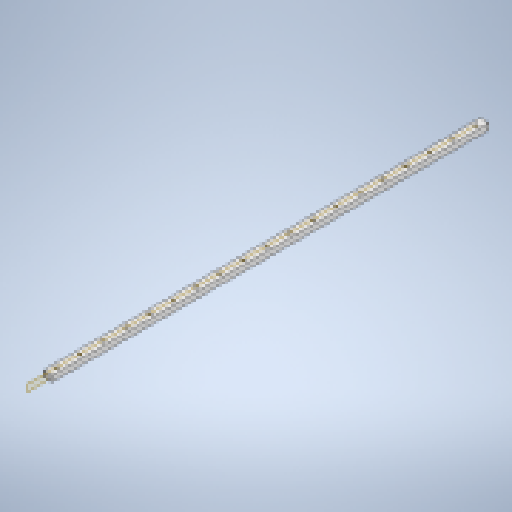
# Autodesk Inventor part: MGN15H-750
Saved by Autodesk Inventor 2023 (Build 270158000, 158)
## iProperties
Created: 2022-04-29
Part Number: MGN15H-750
Material: Generic
Document SubType Name: Modeling
Designer: plebbb
Density: 1 g/cm^3
Appearance: Default
Author: plebbb
Autodesk Inventor part; units mm, degrees
ref_plane "YZ Plane" through (0, 0, 0) normal (1, 0, 0) x (0, 1, 0)
ref_plane "XZ Plane" through (0, 0, 0) normal (0, 1, 0) x (-1, 0, 0)
ref_plane "XY Plane" through (0, 0, 0) normal (0, 0, 1) x (1, 0, 0)
sketch "Sketch1" plane through (0, 0, 0) normal (0, 0, 1) x (1, 0, 0)
  line L0 (0, 0) -> (15, 0)
  line L1 (15, 0) -> (15, 10)
  line L2 (15, 10) -> (0, 10)
  line L3 (0, 10) -> (0, 0)
  dimension "d0" = 15
  dimension "d1" = 10
  constraints: 9 end point, 2 parallel, 1 horizontal, 1 perpendicular
  measures "d0" distance of L0.start L0.end
  measures "d1" distance of L0.end L1.end
extrude "Extrusion1" add sketch "Sketch1" along normal blind 750
ref_plane "Work Plane1" through (7.5, 10, 750) normal (1, 0, 0) x (0, 0, -1)
sketch "Sketch4" plane through (7.5, 10, 750) normal (1, 0, 0) x (0, 0, -1)
  line L0 (732, 0) -> (732, -4.5)
  line L1 (738, -4.5) -> (738, 0)
  line L2 (732, -4.5) -> (733.25, -4.5)
  line L3 (733.25, -4.5) -> (733.25, -10)
  line L4 (733.25, -10) -> (736.75, -10)
  line L5 (736.75, -10) -> (736.75, -4.5)
  line L6 (736.75, -4.5) -> (738, -4.5)
  line L7 (750, 0) -> (0, 0) projected
  line L8 (750, -10) -> (0, -10) projected
  line L9 (732, 0) -> (738, 0)
  line L10 (735, -10) -> (735, 0)
  point P0 (738, -2.25)
  point P1 (735, 0)
  dimension "d6" = 6
  dimension "d7" = 3.5
  dimension "d8" = 4.5
  dimension "d9" = 15
  constraints: 18 end point, 4 perpendicular, 4 point on line, 3 midpoint, 2 collinear, 2 vertical, 1 horizontal
  measures "d6" distance from line of point (738, -2.25) L0
  measures "d7" distance of L3.end L4.end
  measures "d8" distance of L1.start L1.end
  measures "d9" distance of L8.start L10.start
revolve "Revolution1" cut sketch "Sketch4" angle 360 about axis through (7.5, 0, 15) along (0, -1, 0) contours L7 L1 L6 L5 L4 L10
pattern_linear "Rectangular Pattern1" count 20 spacing 40 along (0, 0, 1) of "Revolution1"
body "Solid1"
